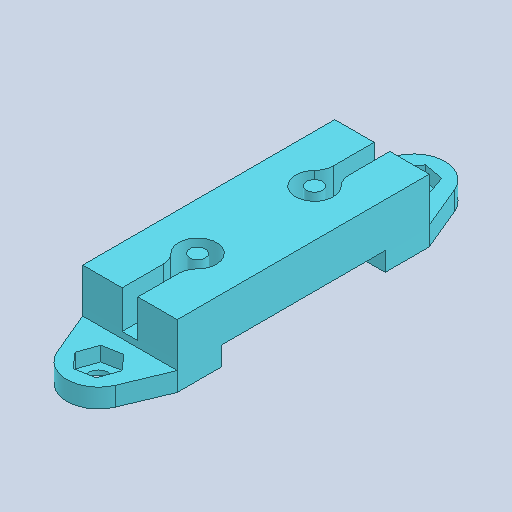
# Autodesk Inventor part: крепление_ремня_новое
Saved by Autodesk Inventor 2023.1 (Build 271208000, 208)
## iProperties
Created: 2026-02-03
Part Number: крепление_ремня_новое
Material: Типовые
Document SubType Name: Modeling
Designer: DELL
Density: 1 g/cm^3
Appearance: Серо-синий
Author: DELL
Autodesk Inventor part; units mm, degrees
ref_plane "YZ Plane" through (0, 0, 0) normal (1, 0, 0) x (0, 1, 0)
ref_plane "XZ Plane" through (0, 0, 0) normal (0, 1, 0) x (-1, 0, 0)
ref_plane "XY Plane" through (0, 0, 0) normal (0, 0, 1) x (1, 0, 0)
sketch "Эскиз1" plane through (0, 0, 0) normal (0, 1, 0) x (-1, 0, 0)
  line L0 (-7.5, 20) -> (7.5, 20)
  line L1 (7.5, 20) -> (7.5, -20)
  line L2 (7.5, -20) -> (-7.5, -20)
  line L3 (-7.5, -20) -> (-7.5, 20)
  line L4 (-7.5, 20) -> (7.5, -20) construction
  line L5 (7.5, 20) -> (-7.5, -20) construction
  line L6 (-1.05, 20) -> (1.05, 20)
  line L7 (1.05, 20) -> (1.05, 10)
  line L8 (1.05, 10) -> (-1.05, 10)
  line L9 (-1.05, 10) -> (-1.05, 20)
  circle A0 centre (0, 7.1898) radius 3
  circle A1 centre (0, 7.1898) radius 2
  point P0 (0, 0)
  point P1 (0, 20)
  dimension "d0" = 40
  dimension "d1" = 15
  dimension "d2" = 2.1
  dimension "d3" = 10
  dimension "d7" = 6
  dimension "d8" = 4
  constraints: 20 end point, 4 midpoint, 4 parallel, 2 centre point, 2 horizontal, 2 perpendicular, 2 point on circle, 1 coincident
  measures "d0" distance of L0.end L1.end
  measures "d1" distance of L0.start L0.end
  measures "d2" distance of L7.end L8.end
  measures "d3" distance of L6.end L7.end
  measures "d7" diameter of A0
  measures "d8" diameter of A1
extrude "Выдавливание1" add sketch "Эскиз1" along normal blind 10 contours L0 L9 A0 L7 L1 L2 L3 | L0 L7 A0 L9 | A0 L8 | L8 A0 | A1
sketch "Эскиз2" plane through (0, 10, 0) normal (0, 1, 0) x (1, 0, 0)
  line L0 (1.25, 20) -> (1.25, 12)
  line L1 (1.25, 12) -> (-1.25, 12)
  line L2 (-1.25, 12) -> (-1.25, 20)
  circle A0 centre (0, 9.2728) radius 3
  circle A1 centre (0, 9.2728) radius 1.25
  line L3 (7.5, -20) -> (7.5, 20) projected
  line L4 (7.5, 20) -> (-7.5, 20) projected
  line L5 (-7.5, 20) -> (-7.5, -20) projected
  line L6 (-7.5, -20) -> (7.5, -20) projected
  line L7 (-1.25, 20) -> (1.25, 20)
  point P0 (0, 20)
  dimension "d13" = 2.5
  dimension "d14" = 8
  dimension "d15" = 6
  dimension "d16" = 2.5
  dimension "d23" = 8
  constraints: 8 end point, 2 centre point, 2 midpoint, 2 point on circle, 1 coincident, 1 horizontal, 1 parallel
  measures "d13" distance of L0.end L1.end
  measures "d14" distance of L0.start L0.end
  measures "d15" diameter of A0
  measures "d16" diameter of A1
  measures "d23" distance of L1.end L2.end
extrude "Выдавливание2" cut sketch "Эскиз2" against normal blind 6 contours L0 A0 L2 L4 | A0 L1 | L1 A0
mirror "Зеркальное отражение1" about plane through (0, 0, 0) normal (0, 0, 1) of "Выдавливание2"
sketch "Эскиз3" plane through (7.5, 0, 20) normal (1, 0, 0) x (0, 0, -1)
  line L0 (7, 3) -> (33, 3)
  line L1 (33, 3) -> (33, 0)
  line L2 (33, 0) -> (7, 0)
  line L3 (7, 0) -> (7, 3)
  line L4 (7, 3) -> (33, 0) construction
  line L5 (33, 3) -> (7, 0) construction
  line L6 (0, 0) -> (40, 0) projected
  point P0 (20, 0)
  point P1 (20, 1.5)
  point P2 (20, 0)
  dimension "d19" = 26
  dimension "d20" = 3
  constraints: 12 end point, 4 midpoint, 2 parallel, 1 horizontal, 1 perpendicular
  measures "d19" distance of L1.end L2.end
  measures "d20" distance of L0.end L1.end
extrude "Выдавливание3" cut sketch "Эскиз3" against normal up to surface (15 mm away)
sketch "Эскиз4" plane through (0, 0, 0) normal (0, -1, 0) x (1, 0, 0)
  circle A0 centre (0, -25) radius 5
  circle A1 centre (0, -25) radius 1.6
  line L0 (7.5, 20) -> (7.5, -20) projected
  line L1 (7.5, -20) -> (4.6154, -26.9231)
  line L2 (-1.25, -20) -> (-7.5, -20) projected
  line L3 (-4.6154, -26.9231) -> (-7.5, -20)
  line L4 (7.5, -20) -> (-7.5, -20) projected
  point P0 (0, 0)
  dimension "d24" = 10
  dimension "d25" = 3.2
  constraints: 4 end point, 3 tangent, 2 centre point, 2 point on circle, 1 coincident, 1 equal length
  measures "d24" diameter of A0
  measures "d25" diameter of A1
extrude "Выдавливание4" add sketch "Эскиз4" against normal blind 3
sketch "Эскиз5" plane through (0, 3, 0) normal (0, 1, 0) x (1, 0, 0)
  circle A0 centre (0, 25) radius 1.6 projected
  arc A1 (4.6154, 26.9231) -> (-4.6154, 26.9231) centre (0, 25) ccw projected
  line L0 (-3.1186, 25.5982) -> (-1.0412, 27.9999)
  line L1 (-1.0412, 27.9999) -> (2.0774, 27.4016)
  line L2 (2.0774, 27.4016) -> (3.1186, 24.4018)
  line L3 (3.1186, 24.4018) -> (1.0412, 22.0001)
  line L4 (1.0412, 22.0001) -> (-2.0774, 22.5984)
  line L5 (-2.0774, 22.5984) -> (-3.1186, 25.5982)
  point P0 (0, 0)
  point P1 (-2.598, 24.0983)
  point P2 (2.598, 25.9017)
  dimension "d32" = 5.5
  constraints: 12 end point, 2 midpoint, 1 coincident, 13 other
  measures "d32" distance between parallel lines of L2 L5
extrude "Выдавливание5" cut sketch "Эскиз5" against normal blind 2.3
mirror "Зеркальное отражение2" about plane through (0, 0, 0) normal (0, 0, 1) of "Выдавливание4", "Выдавливание5"
fillet "Сопряжение1" radius 3 4 edges at (-1.25, 7, -12) (1.25, 7, -12) (-1.25, 7, 12) (1.25, 7, 12)
